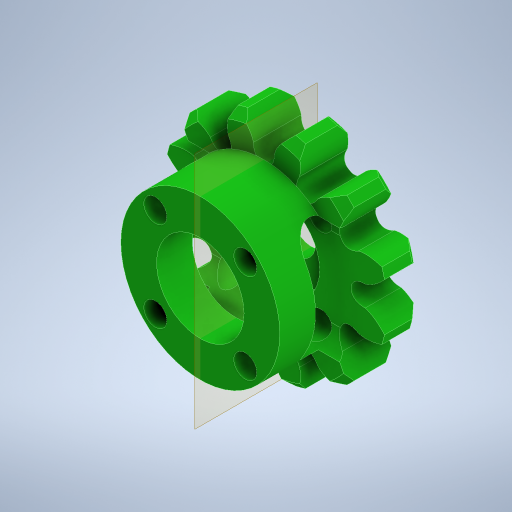
# Autodesk Inventor part: шестерня12-china
Saved by Autodesk Inventor 2024 (Build 280153000, 153)
## iProperties
Created: 2025-10-14
Part Number: шестерня12-china
Material: Generic
Document SubType Name: Modeling
Designer: DELL
Density: 1 g/cm^3
Appearance: Темно-зеленый
Author: DELL
Autodesk Inventor part; units mm, degrees
ref_plane "YZ Plane" through (0, 0, 0) normal (1, 0, 0) x (0, 1, 0)
ref_plane "XZ Plane" through (0, 0, 0) normal (0, 1, 0) x (-1, 0, 0)
ref_plane "XY Plane" through (0, 0, 0) normal (0, 0, 1) x (1, 0, 0)
sketch "Sketch1" plane through (0, 0, 0) normal (0, 0, 1) x (1, 0, 0)
  spline S0 degree 3 poles (-3.0087, 13.6604) (-2.9154, 13.5764) (-2.7289, 13.4085) (-2.4652, 13.1397) (-2.215, 12.8584) (-1.9815, 12.563) (-1.7672, 12.2533) (-1.608, 11.9827) (-1.4953, 11.7584) (-1.42, 11.586) (-1.3534, 11.4097) (-1.324, 11.2876) (-1.3093, 11.2266) knots 0 0 0 0 0.037634 0.075268 0.112902 0.150535 0.188166 0.225794 0.244611 0.263428 0.282243 0.30105 0.30105 0.30105 0.30105
  spline S1 degree 3 poles (-1.3093, 11.2266) (-1.3081, 11.1237) (-1.3062, 10.9693) (-1.2835, 10.7645) (-1.2555, 10.6127) (-1.2209, 10.4621) (-1.1712, 10.3158) (-1.1128, 10.1727) (-1.0388, 10.037) (-0.951, 9.9097) (-0.8483, 9.794) (-0.7312, 9.6929) (-0.6003, 9.6102) (-0.4585, 9.5481) (-0.3086, 9.5088) (-0.1543, 9.4971) (0, 9.5015) (0.1543, 9.4971) (0.3086, 9.5088) (0.4585, 9.5481) (0.6003, 9.6102) (0.7312, 9.6929) (0.8483, 9.794) (0.951, 9.9097) (1.0388, 10.037) (1.1128, 10.1727) (1.1712, 10.3158) (1.2209, 10.4621) (1.2555, 10.6127) (1.2835, 10.7645) (1.3062, 10.9693) (1.3081, 11.1237) (1.3093, 11.2266) knots 0 0 0 0 0.03086 0.046295 0.061729 0.077164 0.092597 0.10803 0.123465 0.138895 0.154322 0.169746 0.185167 0.200585 0.215997 0.231413 0.246848 0.262284 0.2777 0.293112 0.30853 0.323951 0.339375 0.354802 0.370232 0.385667 0.4011 0.416533 0.431968 0.447402 0.462836 0.493697 0.493697 0.493697 0.493697
  spline S2 degree 3 poles (1.3093, 11.2266) (1.324, 11.2876) (1.3534, 11.4097) (1.42, 11.586) (1.4953, 11.7584) (1.608, 11.9827) (1.7672, 12.2533) (1.9815, 12.563) (2.215, 12.8584) (2.4652, 13.1397) (2.7289, 13.4085) (2.9154, 13.5764) (3.0087, 13.6604) knots 0 0 0 0 0.018807 0.037622 0.056439 0.075256 0.112884 0.150515 0.188148 0.225782 0.263416 0.30105 0.30105 0.30105 0.30105
  circle A0 centre (0, 0) radius 9.5 construction
  circle A1 centre (0, 0) radius 11.2763 construction
  circle A2 centre (0, 0) radius 12 construction
  circle A3 centre (0, 0) radius 13.9878
  point P0 (-2.7316, 13.4057)
  point P1 (-2.4675, 13.1376)
  point P2 (-2.2178, 12.856)
  point P3 (-1.9847, 12.5606)
  point P4 (-1.7711, 12.2508)
  point P5 (-1.5811, 11.926)
  point P6 (-1.4968, 11.7577)
  point P7 (-1.4215, 11.5853)
  point P8 (-1.3572, 11.4085)
  point P9 (-1.2988, 10.9182)
  point P10 (-1.2817, 10.7648)
  point P11 (-1.2544, 10.6129)
  point P12 (-1.2184, 10.4628)
  point P13 (-1.1698, 10.3163)
  point P14 (-1.1102, 10.1739)
  point P15 (-1.0365, 10.0384)
  point P16 (-0.9485, 9.9116)
  point P17 (-0.8459, 9.7964)
  point P18 (-0.7288, 9.6959)
  point P19 (-0.5984, 9.6136)
  point P20 (-0.4571, 9.5519)
  point P21 (-0.3079, 9.5134)
  point P22 (-0.1544, 9.4998)
  point P23 (0, 9.5)
  point P24 (0.1544, 9.4998)
  point P25 (0.3079, 9.5134)
  point P26 (0.4571, 9.5519)
  point P27 (0.5984, 9.6136)
  point P28 (0.7288, 9.6959)
  point P29 (0.8459, 9.7964)
  point P30 (0.9485, 9.9116)
  point P31 (1.0365, 10.0384)
  point P32 (1.1102, 10.1739)
  point P33 (1.1698, 10.3163)
  point P34 (1.2184, 10.4628)
  point P35 (1.2544, 10.6129)
  point P36 (1.2817, 10.7648)
  point P37 (1.2988, 10.9182)
  point P38 (1.3572, 11.4085)
  point P39 (1.4215, 11.5853)
  point P40 (1.4968, 11.7577)
  point P41 (1.5811, 11.926)
  point P42 (1.7711, 12.2508)
  point P43 (1.9847, 12.5606)
  point P44 (2.2178, 12.856)
  point P45 (2.4675, 13.1376)
  point P46 (2.7316, 13.4057)
  constraints: 4 centre point, 2 point on circle, 109 other
extrude "Выдавливание1" add sketch "Sketch1" against normal blind 6
extrude "Выдавливание2" cut sketch "Sketch1" against normal blind 10 contours A3 S2 S1 S0 picked at (-0.374, 12.578)
chamfer "Фаска1" distance 1 angle 45 2 edges at (0, -13.9878, 0) (0, -13.9878, -6)
pattern_circular "Круговой массив2" count 12 over 360 about axis through (0, 0, 0) along (0, 0, -1) of "Выдавливание2"
sketch "Эскиз2" plane through (0, 0, 0) normal (0, 0, 1) x (1, 0, 0)
  circle A0 centre (0, 0) radius 10
  dimension "d13" = 20
  constraints: 1 centre point, 1 coincident
  measures "d13" diameter of A0
extrude "Выдавливание3" add sketch "Эскиз2" along normal blind 8
sketch "Эскиз13" plane through (0, 0, 8) normal (0, 0, 1) x (1, 0, 0)
  circle A0 centre (0, 0) radius 8 construction
  line L0 (0, 0) -> (5.6569, 5.6569) construction
  line L1 (0, 0) -> (8, 0) construction
  circle A1 centre (5.6569, 5.6569) radius 1.45
  circle A2 centre (5.6569, -5.6569) radius 1.45
  circle A3 centre (-5.6569, -5.6569) radius 1.45
  circle A4 centre (-5.6569, 5.6569) radius 1.45
  dimension "d65" = 16
  dimension "d66" = 8
  dimension "d67" = 45
  dimension "d68" = 2.9
  dimension "d69" = 2.9
  dimension "d70" = 2.9
  dimension "d71" = 2.9
  constraints: 5 centre point, 4 end point, 3 point on circle, 2 coincident, 1 equal length, 1 horizontal
  measures "d65" diameter of A0
  measures "d66" distance of L0.start L0.end
  measures "d67" angle of L1 L0
  measures "d68" diameter of A1
  measures "d69" diameter of A2
  measures "d70" diameter of A3
  measures "d71" diameter of A4
extrude "Выдавливание13" cut sketch "Эскиз13" against normal blind 14
sketch "Эскиз14" plane through (0, 0, 8) normal (0, 0, 1) x (1, 0, 0)
  circle A0 centre (0, 0) radius 5.5
  dimension "d74" = 11
  constraints: 1 centre point, 1 coincident
  measures "d74" diameter of A0
extrude "Выдавливание14" cut sketch "Эскиз14" against normal blind 12
ref_plane "РабПлоскость4" through (0, 0, 8) normal (1, 0, 0) x (0, 0, -1)
ref_plane "РабПлоскость3" through (5.6569, -5.6569, 8) normal (0.7071, 0.7071, 0) x (0, 0, -1)
sketch "Эскиз15" plane through (0, 0, 8) normal (1, 0, 0) x (0, 0, -1)
  line L0 (12, -5.5) -> (12, 5.5) construction
  line L1 (12, 0) -> (-20.0789, 0) construction
  line L2 (7, 5) -> (7, -5) construction
  line L3 (4.5, 5) -> (4.5, -5)
  line L4 (9.5, -5) -> (9.5, 5)
  arc A0 (9.5, 5) -> (4.5, 5) centre (7, 5) ccw
  arc A1 (4.5, -5) -> (9.5, -5) centre (7, -5) ccw
  line L5 (0, -5.5) -> (0, 5.5) projected
  point P0 (7, 0)
  dimension "d81" = 5
  dimension "d82" = 5
  dimension "d83" = 4.5
  constraints: 10 end point, 4 point on circle, 4 tangent, 2 centre point, 2 midpoint, 1 horizontal, 1 parallel, 1 perpendicular, 1 point on line
  measures "d81" distance of point (7, 0) L2.end
  measures "d82" diameter of A1
  measures "d83" distance between parallel lines of L5 L3
extrude "Выдавливание15" cut sketch "Эскиз15" along normal mid plane 40
sketch "Эскиз16" plane through (0, 0, -4) normal (0, 0, 1) x (1, 0, 0)
  arc A0 (-2.2913, 5) -> (-2.2913, -5) centre (0, 0) ccw projected
  circle A1 centre (0, 0) radius 2.5
  dimension "d86" = 5
  constraints: 1 centre point, 1 coincident
  measures "d86" diameter of A1
extrude "Выдавливание16" cut sketch "Эскиз16" against normal blind 14
equation "\"Модуль\" = 2"
equation "\"Угол_зацепления\" = 20deg"
equation "\"Зазор_профиля_зуба\" = 0.25"
equation "\"Радиус_закругления_зуба\" = 0.35"
equation "\"Диаметр_головки\" = 27.97554"
equation "\"Диаметр_впадин\" = 19"
equation "\"Основной_диаметр\" = 22.55262"
equation "\"Средний_диаметр\" = 24"
equation "\"Коэффициент_смещения\" = 0"
equation "\"Изменение_высоты_головки_зуба\" = 0.006115"
equation "\"Окружной_шаг\" = 6.283185"
equation "\"Общий_сдвиг_инструмента\" = 0"
equation "\"Внутренний\" = 0"
